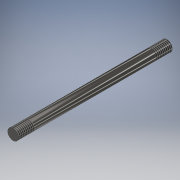
# Autodesk Inventor part: shaft test
Saved by Autodesk Inventor 2018 (Build 220112000, 112)
## iProperties
Created: 2017-09-19
Part Number: shaft test
Material: Generic
Document SubType Name: Modeling
Designer: M227958
Density: 1 g/cm^3
Appearance: Chrome - Polished Black
Author: M227958
Autodesk Inventor part; units mm, degrees
ref_plane "YZ Plane" through (0, 0, 0) normal (1, 0, 0) x (0, 1, 0)
ref_plane "XZ Plane" through (0, 0, 0) normal (0, 1, 0) x (-1, 0, 0)
ref_plane "XY Plane" through (0, 0, 0) normal (0, 0, 1) x (1, 0, 0)
sketch "Sketch2" plane through (0, 0, 0) normal (0, 1, 0) x (-1, 0, 0)
  circle A0 centre (0, 0) radius 4
  dimension "d7" = 8
  constraints: 1 centre point, 1 coincident
  measures "d7" diameter of A0
extrude "Extrusion2" add sketch "Sketch2" along normal blind 113.733
thread "Thread3" size "M8x1.25" class "6g" standard "ANSI Metric M Profile" length 12
thread "Thread4" size "M8x1.25" class "6g" standard "ANSI Metric M Profile" length 12
body "Solid2"
